Autodesk Fusion 360 part; units mm, degrees
(part 3 of 4)
sketch "Sketch9" plane through (0, 17, 0) normal (0, 1, 0) x (-1, 0, 0)
  line L0 (-96.2371, 19.0203) -> (-96.2371, 18.4195)
  line L1 (-96.2371, 18.4195) -> (-95.4378, 18.4195)
  line L2 (-95.4378, 18.4195) -> (-95.4378, 5.6203)
  line L3 (-95.4378, 5.6203) -> (-96.2371, 5.6203)
  line L4 (-96.2371, 5.6203) -> (-96.2371, 5.0195)
  line L5 (-96.2371, 5.0195) -> (-110.23659, 5.0195)
  line L6 (-110.23659, 5.0195) -> (-110.23659, 5.6203)
  line L7 (-110.23659, 5.6203) -> (-111.03722, 5.6203)
  line L8 (-111.03722, 5.6203) -> (-111.03722, 18.4195)
  line L9 (-111.03722, 18.4195) -> (-110.23659, 18.4195)
  line L10 (-110.23659, 18.4195) -> (-110.23659, 19.0203)
  line L11 (-110.23659, 19.0203) -> (-96.2371, 19.0203)
  line L12 (-31.1441, 18.4195) -> (-31.1441, 5.6203)
  line L13 (-31.1441, 5.6203) -> (-31.9449, 5.6203)
  line L14 (-31.9449, 5.6203) -> (-31.9449, 5.0195)
  line L15 (-31.9449, 5.0195) -> (-45.9442, 5.0195)
  line L16 (-45.9442, 5.0195) -> (-45.9442, 5.6203)
  line L17 (-45.9442, 5.6203) -> (-46.745, 5.6203)
  line L18 (-46.745, 5.6203) -> (-46.745, 18.4195)
  line L19 (-46.745, 18.4195) -> (-45.9442, 18.4195)
  line L20 (-45.9442, 18.4195) -> (-45.9442, 19.0203)
  line L21 (-45.9442, 19.0203) -> (-31.9449, 19.0203)
  line L22 (-31.9449, 19.0203) -> (-31.9449, 18.4195)
  line L23 (-31.9449, 18.4195) -> (-31.1441, 18.4195)
  line L24 (-21.6191, 24.6704) -> (-22.4199, 24.6704)
  line L25 (-22.4199, 24.6704) -> (-22.4199, 24.0696)
  line L26 (-22.4199, 24.0696) -> (-36.4192, 24.0696)
  line L27 (-36.4192, 24.0696) -> (-36.4192, 24.6704)
  line L28 (-36.4192, 24.6704) -> (-37.2186, 24.6704)
  line L29 (-37.2186, 24.6704) -> (-37.2186, 37.4695)
  line L30 (-37.2186, 37.4695) -> (-36.4192, 37.4695)
  line L31 (-36.4192, 37.4695) -> (-36.4192, 38.0703)
  line L32 (-36.4192, 38.0703) -> (-22.4199, 38.0703)
  line L33 (-22.4199, 38.0703) -> (-22.4199, 37.4695)
  line L34 (-22.4199, 37.4695) -> (-21.6191, 37.4695)
  line L35 (-21.6191, 37.4695) -> (-21.6191, 24.6704)
  line L36 (-62.6115, -0.0297) -> (-46.391293, -0.0297)
  line L37 (-46.391293, -0.0297) -> (-46.391293, -0.6305)
  line L38 (-46.391293, -0.6305) -> (-45.592293, -0.6305)
  line L39 (-45.592293, -0.6305) -> (-45.592293, -3.205101)
  line L40 (-45.592293, -3.205101) -> (-43.156293, -3.205101)
  arc A0 (-43.156293, -8.205101) -> (-43.156293, -3.205101) centre (-43.156293, -5.705101) ccw
  line L41 (-43.156293, -8.205101) -> (-45.592293, -8.205101)
  line L42 (-45.592293, -8.205101) -> (-45.592293, -13.42971)
  line L43 (-45.592293, -13.42971) -> (-46.391293, -13.42971)
  line L44 (-46.391293, -13.42971) -> (-46.391293, -14.03054)
  line L45 (-46.391293, -14.03054) -> (-62.6115, -14.03054)
  line L46 (-62.6115, -14.03054) -> (-62.6115, -13.42971)
  line L47 (-62.6115, -13.42971) -> (-63.4123, -13.42971)
  line L48 (-63.4123, -13.42971) -> (-63.4123, -0.6305)
  line L49 (-63.4123, -0.6305) -> (-62.6115, -0.6305)
  line L50 (-62.6115, -0.6305) -> (-62.6115, -0.0297)
  circle A1 centre (-90.056293, 5.844899) radius 2.5
  line L51 (-100.2003, -13.42971) -> (-100.9996, -13.42971)
  line L52 (-100.9996, -13.42971) -> (-100.9996, -14.03054)
  line L53 (-100.9996, -14.03054) -> (-115.00047, -14.03054)
  line L54 (-115.00047, -14.03054) -> (-115.00047, -14)
  line L55 (-115.00047, -14) -> (-117.382293, -14)
  line L56 (-117.382293, -14) -> (-117.382293, -13.42971)
  line L57 (-117.382293, -13.42971) -> (-118.181293, -13.42971)
  line L58 (-118.181293, -13.42971) -> (-118.181293, -0.6305)
  line L59 (-118.181293, -0.6305) -> (-117.382293, -0.6305)
  line L60 (-117.382293, -0.6305) -> (-117.382293, -0.0297)
  line L61 (-117.382293, -0.0297) -> (-100.9996, -0.0297)
  line L62 (-100.9996, -0.0297) -> (-100.9996, -0.6305)
  line L63 (-100.9996, -0.6305) -> (-100.2003, -0.6305)
  line L64 (-100.2003, -0.6305) -> (-100.2003, -13.42971)
  line L65 (120.457, 5.6203) -> (120.457, 5.0195)
  line L66 (120.457, 5.0195) -> (106.457, 5.0195)
  line L67 (106.457, 5.0195) -> (106.457, 5.6203)
  line L68 (106.457, 5.6203) -> (105.656, 5.6203)
  line L69 (105.656, 5.6203) -> (105.656, 18.4195)
  line L70 (105.656, 18.4195) -> (106.457, 18.4195)
  line L71 (106.457, 18.4195) -> (106.457, 19.0203)
  line L72 (106.457, 19.0203) -> (120.457, 19.0203)
  line L73 (120.457, 19.0203) -> (120.457, 18.4195)
  line L74 (120.457, 18.4195) -> (121.257, 18.4195)
  line L75 (121.257, 18.4195) -> (121.257, 5.6203)
  line L76 (121.257, 5.6203) -> (120.457, 5.6203)
  circle A2 centre (62.431, -5.905101) radius 2.5
  line L77 (99.313, 57.1203) -> (113.313, 57.1203)
  line L78 (113.313, 57.1203) -> (113.313, 56.5195)
  line L79 (113.313, 56.5195) -> (114.112, 56.5195)
  line L80 (114.112, 56.5195) -> (114.112, 43.7204)
  line L81 (114.112, 43.7204) -> (113.313, 43.7204)
  line L82 (113.313, 43.7204) -> (113.313, 43.1196)
  line L83 (113.313, 43.1196) -> (99.313, 43.1196)
  line L84 (99.313, 43.1196) -> (99.313, 43.7204)
  line L85 (99.313, 43.7204) -> (98.513, 43.7204)
  line L86 (98.513, 43.7204) -> (98.513, 56.5195)
  line L87 (98.513, 56.5195) -> (99.313, 56.5195)
  line L88 (99.313, 56.5195) -> (99.313, 57.1203)
  line L89 (101.693, 24.0696) -> (101.693, 24.6704)
  line L90 (101.693, 24.6704) -> (100.894, 24.6704)
  line L91 (100.894, 24.6704) -> (100.894, 37.4695)
  line L92 (100.894, 37.4695) -> (101.693, 37.4695)
  line L93 (101.693, 37.4695) -> (101.693, 38.0703)
  line L94 (101.693, 38.0703) -> (115.694, 38.0703)
  line L95 (115.694, 38.0703) -> (115.694, 37.4695)
  line L96 (115.694, 37.4695) -> (116.493, 37.4695)
  line L97 (116.493, 37.4695) -> (116.493, 24.6704)
  line L98 (116.493, 24.6704) -> (115.694, 24.6704)
  line L99 (115.694, 24.6704) -> (115.694, 24.0696)
  line L100 (115.694, 24.0696) -> (101.693, 24.0696)
  line L101 (87.119, 56.5195) -> (87.918, 56.5195)
  line L102 (87.918, 56.5195) -> (87.918, 43.7204)
  line L103 (87.918, 43.7204) -> (87.119, 43.7204)
  line L104 (87.119, 43.7204) -> (87.119, 43.1196)
  line L105 (87.119, 43.1196) -> (73.118, 43.1196)
  line L106 (73.118, 43.1196) -> (73.118, 43.7204)
  line L107 (73.118, 43.7204) -> (72.319, 43.7204)
  line L108 (72.319, 43.7204) -> (72.319, 56.5195)
  line L109 (72.319, 56.5195) -> (73.118, 56.5195)
  line L110 (73.118, 56.5195) -> (73.118, 57.1203)
  line L111 (73.118, 57.1203) -> (87.119, 57.1203)
  line L112 (87.119, 57.1203) -> (87.119, 56.5195)
  line L113 (87.407, 5.0195) -> (87.407, 5.6203)
  line L114 (87.407, 5.6203) -> (86.606, 5.6203)
  line L115 (86.606, 5.6203) -> (86.606, 18.4195)
  line L116 (86.606, 18.4195) -> (87.407, 18.4195)
  line L117 (87.407, 18.4195) -> (87.407, 19.0203)
  line L118 (87.407, 19.0203) -> (101.407, 19.0203)
  line L119 (101.407, 19.0203) -> (101.407, 18.4195)
  line L120 (101.407, 18.4195) -> (102.207, 18.4195)
  line L121 (102.207, 18.4195) -> (102.207, 5.6203)
  line L122 (102.207, 5.6203) -> (101.407, 5.6203)
  line L123 (101.407, 5.6203) -> (101.407, 5.0195)
  line L124 (101.407, 5.0195) -> (87.407, 5.0195)
  line L125 (77.882, 24.6704) -> (77.081, 24.6704)
  line L126 (77.081, 24.6704) -> (77.081, 37.4695)
  line L127 (77.081, 37.4695) -> (77.882, 37.4695)
  line L128 (77.882, 37.4695) -> (77.882, 38.0703)
  line L129 (77.882, 38.0703) -> (91.882, 38.0703)
  line L130 (91.882, 38.0703) -> (91.882, 37.4695)
  line L131 (91.882, 37.4695) -> (92.682, 37.4695)
  line L132 (92.682, 37.4695) -> (92.682, 24.6704)
  line L133 (92.682, 24.6704) -> (91.882, 24.6704)
  line L134 (91.882, 24.6704) -> (91.882, 24.0696)
  line L135 (91.882, 24.0696) -> (77.882, 24.0696)
  line L136 (77.882, 24.0696) -> (77.882, 24.6704)
  circle A3 centre (90.731, 42.8948) radius 2.5
  line L137 (121.257, -0.6305) -> (121.257, -13.42971)
  line L138 (121.257, -13.42971) -> (120.457, -13.42971)
  line L139 (120.457, -13.42971) -> (120.457, -14.03054)
  line L140 (120.457, -14.03054) -> (106.457, -14.03054)
  line L141 (106.457, -14.03054) -> (106.457, -14)
  line L142 (106.457, -14) -> (101.407, -14)
  line L143 (101.407, -14) -> (101.407, -14.03054)
  line L144 (101.407, -14.03054) -> (87.407, -14.03054)
  line L145 (87.407, -14.03054) -> (87.407, -13.42971)
  line L146 (87.407, -13.42971) -> (86.606, -13.42971)
  line L147 (86.606, -13.42971) -> (86.606, -0.6305)
  line L148 (86.606, -0.6305) -> (87.407, -0.6305)
  line L149 (87.407, -0.6305) -> (87.407, -0.0297)
  line L150 (87.407, -0.0297) -> (120.457, -0.0297)
  line L151 (120.457, -0.0297) -> (120.457, -0.6305)
  line L152 (120.457, -0.6305) -> (121.257, -0.6305)
  line L153 (41.363, -0.6305) -> (42.162, -0.6305)
  line L154 (42.162, -0.6305) -> (42.162, -0.0297)
  line L155 (42.162, -0.0297) -> (58.544, -0.0297)
  line L156 (58.544, -0.0297) -> (58.544, -0.6305)
  line L157 (58.544, -0.6305) -> (59.343, -0.6305)
  line L158 (59.343, -0.6305) -> (59.343, -13.42971)
  line L159 (59.343, -13.42971) -> (58.544, -13.42971)
  line L160 (58.544, -13.42971) -> (58.544, -14.03054)
  line L161 (58.544, -14.03054) -> (44.543, -14.03054)
  line L162 (44.543, -14.03054) -> (44.543, -14)
  line L163 (44.543, -14) -> (42.162, -14)
  line L164 (42.162, -14) -> (42.162, -13.42971)
  line L165 (42.162, -13.42971) -> (41.363, -13.42971)
  line L166 (41.363, -13.42971) -> (41.363, -0.6305)
  line L167 (25.205, 18.4195) -> (26.006, 18.4195)
  line L168 (26.006, 18.4195) -> (26.006, 5.6203)
  line L169 (26.006, 5.6203) -> (25.205, 5.6203)
  line L170 (25.205, 5.6203) -> (25.205, 5.0195)
  line L171 (25.205, 5.0195) -> (11.206, 5.0195)
  line L172 (11.206, 5.0195) -> (11.206, 5.6203)
  line L173 (11.206, 5.6203) -> (10.405, 5.6203)
  line L174 (10.405, 5.6203) -> (10.405, 18.4195)
  line L175 (10.405, 18.4195) -> (11.206, 18.4195)
  line L176 (11.206, 18.4195) -> (11.206, 19.0203)
  line L177 (11.206, 19.0203) -> (17.022586, 19.0203)
  line L178 (17.022586, 19.0203) -> (17.022586, 19.279382)
  arc A4 (19.339414, 19.279382) -> (17.022586, 19.279382) centre (18.181, 21.4948) ccw
  line L179 (19.339414, 19.279382) -> (19.339414, 19.0203)
  line L180 (19.339414, 19.0203) -> (25.205, 19.0203)
  line L181 (25.205, 19.0203) -> (25.205, 18.4195)
  line L182 (-100.2003, 24.6704) -> (-100.9996, 24.6704)
  line L183 (-100.9996, 24.6704) -> (-100.9996, 24.0696)
  line L184 (-100.9996, 24.0696) -> (-115.00047, 24.0696)
  line L185 (-115.00047, 24.0696) -> (-115.00047, 24.6704)
  line L186 (-115.00047, 24.6704) -> (-115.79972, 24.6704)
  line L187 (-115.79972, 24.6704) -> (-115.79972, 37.4695)
  line L188 (-115.79972, 37.4695) -> (-115.00047, 37.4695)
  line L189 (-115.00047, 37.4695) -> (-115.00047, 38.0703)
  line L190 (-115.00047, 38.0703) -> (-100.9996, 38.0703)
  line L191 (-100.9996, 38.0703) -> (-100.9996, 37.4695)
  line L192 (-100.9996, 37.4695) -> (-100.2003, 37.4695)
  line L193 (-100.2003, 37.4695) -> (-100.2003, 24.6704)
  line L194 (-102.5816, 43.7204) -> (-103.3808, 43.7204)
  line L195 (-103.3808, 43.7204) -> (-103.3808, 43.1196)
  line L196 (-103.3808, 43.1196) -> (-117.38173, 43.1196)
  line L197 (-117.38173, 43.1196) -> (-117.38173, 43.7204)
  line L198 (-117.38173, 43.7204) -> (-118.18099, 43.7204)
  line L199 (-118.18099, 43.7204) -> (-118.18099, 56.5195)
  line L200 (-118.18099, 56.5195) -> (-117.38173, 56.5195)
  line L201 (-117.38173, 56.5195) -> (-117.38173, 57.1203)
  line L202 (-117.38173, 57.1203) -> (-103.3808, 57.1203)
  line L203 (-103.3808, 57.1203) -> (-103.3808, 56.5195)
  line L204 (-103.3808, 56.5195) -> (-102.5816, 56.5195)
  line L205 (-102.5816, 56.5195) -> (-102.5816, 43.7204)
  line L206 (-98.372293, -13.42971) -> (-99.171293, -13.42971)
  line L207 (-99.171293, -13.42971) -> (-99.171293, -0.6305)
  line L208 (-99.171293, -0.6305) -> (-98.372293, -0.6305)
  line L209 (-98.372293, -0.6305) -> (-98.372293, 0)
  line L210 (-98.372293, 0) -> (-65.401293, 0)
  line L211 (-65.401293, 0) -> (-65.401293, -0.6305)
  line L212 (-65.401293, -0.6305) -> (-64.602293, -0.6305)
  line L213 (-64.602293, -0.6305) -> (-64.602293, -13.42971)
  line L214 (-64.602293, -13.42971) -> (-65.401293, -13.42971)
  line L215 (-65.401293, -13.42971) -> (-65.401293, -14.03054)
  line L216 (-65.401293, -14.03054) -> (-98.372293, -14.03054)
  line L217 (-98.372293, -14.03054) -> (-98.372293, -13.42971)
  line L218 (-60.5185, 38.0703) -> (-60.5185, 37.4695)
  line L219 (-60.5185, 37.4695) -> (-59.7177, 37.4695)
  line L220 (-59.7177, 37.4695) -> (-59.7177, 24.6704)
  line L221 (-59.7177, 24.6704) -> (-60.5185, 24.6704)
  line L222 (-60.5185, 24.6704) -> (-60.5185, 24.0696)
  line L223 (-60.5185, 24.0696) -> (-74.5178, 24.0696)
  line L224 (-74.5178, 24.0696) -> (-74.5178, 24.6704)
  line L225 (-74.5178, 24.6704) -> (-75.3186, 24.6704)
  line L226 (-75.3186, 24.6704) -> (-75.3186, 37.4695)
  line L227 (-75.3186, 37.4695) -> (-74.5178, 37.4695)
  line L228 (-74.5178, 37.4695) -> (-74.5178, 38.0703)
  line L229 (-74.5178, 38.0703) -> (-60.5185, 38.0703)
  line L230 (-87.582873, 38.0703) -> (-79.5699, 38.0703)
  line L231 (-79.5699, 38.0703) -> (-79.5699, 37.4695)
  line L232 (-79.5699, 37.4695) -> (-78.7691, 37.4695)
  line L233 (-78.7691, 37.4695) -> (-78.7691, 24.6704)
  line L234 (-78.7691, 24.6704) -> (-79.5699, 24.6704)
  line L235 (-79.5699, 24.6704) -> (-79.5699, 24.0696)
  line L236 (-79.5699, 24.0696) -> (-93.5692, 24.0696)
  line L237 (-93.5692, 24.0696) -> (-93.5692, 24.6704)
  line L238 (-93.5692, 24.6704) -> (-94.3699, 24.6704)
  line L239 (-94.3699, 24.6704) -> (-94.3699, 37.4695)
  line L240 (-94.3699, 37.4695) -> (-93.5692, 37.4695)
  line L241 (-93.5692, 37.4695) -> (-93.5692, 38.0703)
  line L242 (-93.5692, 38.0703) -> (-89.429714, 38.0703)
  line L243 (-89.429714, 38.0703) -> (-89.429714, 38.271592)
  arc A5 (-89.429714, 42.918008) -> (-89.429714, 38.271592) centre (-88.506293, 40.5948) ccw
  line L244 (-89.429714, 42.918008) -> (-89.429714, 43.1196)
  line L245 (-89.429714, 43.1196) -> (-98.3317, 43.1196)
  line L246 (-98.3317, 43.1196) -> (-98.3317, 43.7204)
  line L247 (-98.3317, 43.7204) -> (-99.131, 43.7204)
  line L248 (-99.131, 43.7204) -> (-99.131, 56.5195)
  line L249 (-99.131, 56.5195) -> (-98.3317, 56.5195)
  line L250 (-98.3317, 56.5195) -> (-98.3317, 57.1203)
  line L251 (-98.3317, 57.1203) -> (-84.331, 57.1203)
  line L252 (-84.331, 57.1203) -> (-84.331, 56.5195)
  line L253 (-84.331, 56.5195) -> (-83.5316, 56.5195)
  line L254 (-83.5316, 56.5195) -> (-83.5316, 43.7204)
  line L255 (-83.5316, 43.7204) -> (-84.331, 43.7204)
  line L256 (-84.331, 43.7204) -> (-84.331, 43.1196)
  line L257 (-84.331, 43.1196) -> (-87.582873, 43.1196)
  line L258 (-87.582873, 43.1196) -> (-87.582873, 42.918008)
  arc A6 (-87.582873, 38.271592) -> (-87.582873, 42.918008) centre (-88.506293, 40.5948) ccw
  line L259 (-87.582873, 38.271592) -> (-87.582873, 38.0703)
  line L260 (-27.695, 5.6203) -> (-27.695, 18.4195)
  line L261 (-27.695, 18.4195) -> (-26.8942, 18.4195)
  line L262 (-26.8942, 18.4195) -> (-26.8942, 19.0203)
  line L263 (-26.8942, 19.0203) -> (-12.895, 19.0203)
  line L264 (-12.895, 19.0203) -> (-12.895, 18.4195)
  line L265 (-12.895, 18.4195) -> (-12.094, 18.4195)
  line L266 (-12.094, 18.4195) -> (-12.094, 5.6203)
  line L267 (-12.094, 5.6203) -> (-12.895, 5.6203)
  line L268 (-12.895, 5.6203) -> (-12.895, 5.0195)
  line L269 (-12.895, 5.0195) -> (-26.8942, 5.0195)
  line L270 (-26.8942, 5.0195) -> (-26.8942, 5.6203)
  line L271 (-26.8942, 5.6203) -> (-27.695, 5.6203)
  arc A7 (-13.437968, 42.823995) -> (-13.437968, 38.365605) centre (-12.306293, 40.5948) ccw
  line L272 (-13.437968, 42.823995) -> (-13.437968, 43.1196)
  line L273 (-13.437968, 43.1196) -> (-22.1317, 43.1196)
  line L274 (-22.1317, 43.1196) -> (-22.1317, 43.7204)
  line L275 (-22.1317, 43.7204) -> (-22.9311, 43.7204)
  line L276 (-22.9311, 43.7204) -> (-22.9311, 56.5195)
  line L277 (-22.9311, 56.5195) -> (-22.1317, 56.5195)
  line L278 (-22.1317, 56.5195) -> (-22.1317, 57.1203)
  line L279 (-22.1317, 57.1203) -> (-8.131, 57.1203)
  line L280 (-8.131, 57.1203) -> (-8.131, 56.5195)
  line L281 (-8.131, 56.5195) -> (-7.332, 56.5195)
  line L282 (-7.332, 56.5195) -> (-7.332, 43.7204)
  line L283 (-7.332, 43.7204) -> (-8.131, 43.7204)
  line L284 (-8.131, 43.7204) -> (-8.131, 43.1196)
  line L285 (-8.131, 43.1196) -> (-11.174619, 43.1196)
  line L286 (-11.174619, 43.1196) -> (-11.174619, 42.823995)
  arc A8 (-11.174619, 38.365605) -> (-11.174619, 42.823995) centre (-12.306293, 40.5948) ccw
  line L287 (-11.174619, 38.365605) -> (-11.174619, 38.0703)
  line L288 (-11.174619, 38.0703) -> (-3.37, 38.0703)
  line L289 (-3.37, 38.0703) -> (-3.37, 37.4695)
  line L290 (-3.37, 37.4695) -> (-2.569, 37.4695)
  line L291 (-2.569, 37.4695) -> (-2.569, 24.6704)
  line L292 (-2.569, 24.6704) -> (-3.37, 24.6704)
  line L293 (-3.37, 24.6704) -> (-3.37, 24.0696)
  line L294 (-3.37, 24.0696) -> (-17.369, 24.0696)
  line L295 (-17.369, 24.0696) -> (-17.369, 24.6704)
  line L296 (-17.369, 24.6704) -> (-18.17, 24.6704)
  line L297 (-18.17, 24.6704) -> (-18.17, 37.4695)
  line L298 (-18.17, 37.4695) -> (-17.369, 37.4695)
  line L299 (-17.369, 37.4695) -> (-17.369, 38.0703)
  line L300 (-17.369, 38.0703) -> (-13.437968, 38.0703)
  line L301 (-13.437968, 38.0703) -> (-13.437968, 38.365605)
  line L302 (68.069, 56.5195) -> (68.868, 56.5195)
  line L303 (68.868, 56.5195) -> (68.868, 43.7204)
  line L304 (68.868, 43.7204) -> (68.069, 43.7204)
  line L305 (68.069, 43.7204) -> (68.069, 43.1196)
  line L306 (68.069, 43.1196) -> (54.068, 43.1196)
  line L307 (54.068, 43.1196) -> (54.068, 43.7204)
  line L308 (54.068, 43.7204) -> (53.269, 43.7204)
  line L309 (53.269, 43.7204) -> (53.269, 56.5195)
  line L310 (53.269, 56.5195) -> (54.068, 56.5195)
  line L311 (54.068, 56.5195) -> (54.068, 57.1203)
  line L312 (54.068, 57.1203) -> (68.069, 57.1203)
  line L313 (68.069, 57.1203) -> (68.069, 56.5195)
  line L314 (67.556, -0.6305) -> (68.357, -0.6305)
  line L315 (68.357, -0.6305) -> (68.357, -0.0297)
  line L316 (68.357, -0.0297) -> (82.357, -0.0297)
  line L317 (82.357, -0.0297) -> (82.357, -0.6305)
  line L318 (82.357, -0.6305) -> (83.157, -0.6305)
  line L319 (83.157, -0.6305) -> (83.157, -13.42971)
  line L320 (83.157, -13.42971) -> (82.357, -13.42971)
  line L321 (82.357, -13.42971) -> (82.357, -14.03054)
  line L322 (82.357, -14.03054) -> (68.357, -14.03054)
  line L323 (68.357, -14.03054) -> (68.357, -13.42971)
  line L324 (68.357, -13.42971) -> (67.556, -13.42971)
  line L325 (67.556, -13.42971) -> (67.556, -0.6305)
  line L326 (68.357, 5.0195) -> (68.357, 5.6203)
  line L327 (68.357, 5.6203) -> (67.556, 5.6203)
  line L328 (67.556, 5.6203) -> (67.556, 18.4195)
  line L329 (67.556, 18.4195) -> (68.357, 18.4195)
  line L330 (68.357, 18.4195) -> (68.357, 19.0203)
  line L331 (68.357, 19.0203) -> (82.357, 19.0203)
  line L332 (82.357, 19.0203) -> (82.357, 18.4195)
  line L333 (82.357, 18.4195) -> (83.157, 18.4195)
  line L334 (83.157, 18.4195) -> (83.157, 5.6203)
  line L335 (83.157, 5.6203) -> (82.357, 5.6203)
  line L336 (82.357, 5.6203) -> (82.357, 5.0195)
  line L337 (82.357, 5.0195) -> (68.357, 5.0195)
  line L338 (-79.2817, 56.5195) -> (-79.2817, 57.1203)
  line L339 (-79.2817, 57.1203) -> (-65.281, 57.1203)
  line L340 (-65.281, 57.1203) -> (-65.281, 56.5195)
  line L341 (-65.281, 56.5195) -> (-64.4816, 56.5195)
  line L342 (-64.4816, 56.5195) -> (-64.4816, 43.7204)
  line L343 (-64.4816, 43.7204) -> (-65.281, 43.7204)
  line L344 (-65.281, 43.7204) -> (-65.281, 43.1196)
  line L345 (-65.281, 43.1196) -> (-79.2817, 43.1196)
  line L346 (-79.2817, 43.1196) -> (-79.2817, 43.7204)
  line L347 (-79.2817, 43.7204) -> (-80.0811, 43.7204)
  line L348 (-80.0811, 43.7204) -> (-80.0811, 56.5195)
  line L349 (-80.0811, 56.5195) -> (-79.2817, 56.5195)
  line L350 (-70.0449, 5.0195) -> (-84.0442, 5.0195)
  line L351 (-84.0442, 5.0195) -> (-84.0442, 5.6203)
  line L352 (-84.0442, 5.6203) -> (-84.8449, 5.6203)
  line L353 (-84.8449, 5.6203) -> (-84.8449, 18.4195)
  line L354 (-84.8449, 18.4195) -> (-84.0442, 18.4195)
  line L355 (-84.0442, 18.4195) -> (-84.0442, 19.0203)
  line L356 (-84.0442, 19.0203) -> (-70.0449, 19.0203)
  line L357 (-70.0449, 19.0203) -> (-70.0449, 18.4195)
  line L358 (-70.0449, 18.4195) -> (-69.2441, 18.4195)
  line L359 (-69.2441, 18.4195) -> (-69.2441, 5.6203)
  line L360 (-69.2441, 5.6203) -> (-70.0449, 5.6203)
  line L361 (-70.0449, 5.6203) -> (-70.0449, 5.0195)
  line L362 (-50.1941, 5.6203) -> (-50.9949, 5.6203)
  line L363 (-50.9949, 5.6203) -> (-50.9949, 5.0195)
  line L364 (-50.9949, 5.0195) -> (-64.9942, 5.0195)
  line L365 (-64.9942, 5.0195) -> (-64.9942, 5.6203)
  line L366 (-64.9942, 5.6203) -> (-65.795, 5.6203)
  line L367 (-65.795, 5.6203) -> (-65.795, 18.4195)
  line L368 (-65.795, 18.4195) -> (-64.9942, 18.4195)
  line L369 (-64.9942, 18.4195) -> (-64.9942, 19.0203)
  line L370 (-64.9942, 19.0203) -> (-50.9949, 19.0203)
  line L371 (-50.9949, 19.0203) -> (-50.9949, 18.4195)
  line L372 (-50.9949, 18.4195) -> (-50.1941, 18.4195)
  line L373 (-50.1941, 18.4195) -> (-50.1941, 5.6203)
  line L374 (35.532, 37.4695) -> (35.532, 24.6704)
  line L375 (35.532, 24.6704) -> (34.732, 24.6704)
  line L376 (34.732, 24.6704) -> (34.732, 24.0696)
  line L377 (34.732, 24.0696) -> (20.732, 24.0696)
  line L378 (20.732, 24.0696) -> (20.732, 24.6704)
  line L379 (20.732, 24.6704) -> (19.931, 24.6704)
  line L380 (19.931, 24.6704) -> (19.931, 37.4695)
  line L381 (19.931, 37.4695) -> (20.732, 37.4695)
  line L382 (20.732, 37.4695) -> (20.732, 38.0703)
  line L383 (20.732, 38.0703) -> (34.732, 38.0703)
  line L384 (34.732, 38.0703) -> (34.732, 37.4695)
  line L385 (34.732, 37.4695) -> (35.532, 37.4695)
  line L386 (15.682, 38.0703) -> (15.682, 37.4695)
  line L387 (15.682, 37.4695) -> (16.482, 37.4695)
  line L388 (16.482, 37.4695) -> (16.482, 24.6704)
  line L389 (16.482, 24.6704) -> (15.682, 24.6704)
  line L390 (15.682, 24.6704) -> (15.682, 24.0696)
  line L391 (15.682, 24.0696) -> (1.682, 24.0696)
  line L392 (1.682, 24.0696) -> (1.682, 24.6704)
  line L393 (1.682, 24.6704) -> (0.881, 24.6704)
  line L394 (0.881, 24.6704) -> (0.881, 37.4695)
  line L395 (0.881, 37.4695) -> (1.682, 37.4695)
  line L396 (1.682, 37.4695) -> (1.682, 38.0703)
  line L397 (1.682, 38.0703) -> (15.682, 38.0703)
  line L398 (-61.0311, 56.5195) -> (-60.2317, 56.5195)
  line L399 (-60.2317, 56.5195) -> (-60.2317, 57.1203)
  line L400 (-60.2317, 57.1203) -> (-46.231, 57.1203)
  line L401 (-46.231, 57.1203) -> (-46.231, 56.5195)
  line L402 (-46.231, 56.5195) -> (-45.4316, 56.5195)
  line L403 (-45.4316, 56.5195) -> (-45.4316, 43.7204)
  line L404 (-45.4316, 43.7204) -> (-46.231, 43.7204)
  line L405 (-46.231, 43.7204) -> (-46.231, 43.1196)
  line L406 (-46.231, 43.1196) -> (-60.2317, 43.1196)
  line L407 (-60.2317, 43.1196) -> (-60.2317, 43.7204)
  line L408 (-60.2317, 43.7204) -> (-61.0311, 43.7204)
  line L409 (-61.0311, 43.7204) -> (-61.0311, 56.5195)
  line L410 (10.919, 43.7204) -> (10.919, 43.1196)
  line L411 (10.919, 43.1196) -> (-3.082, 43.1196)
  line L412 (-3.082, 43.1196) -> (-3.082, 43.7204)
  line L413 (-3.082, 43.7204) -> (-3.881, 43.7204)
  line L414 (-3.881, 43.7204) -> (-3.881, 56.5195)
  line L415 (-3.881, 56.5195) -> (-3.082, 56.5195)
  line L416 (-3.082, 56.5195) -> (-3.082, 57.1203)
  line L417 (-3.082, 57.1203) -> (10.919, 57.1203)
  line L418 (10.919, 57.1203) -> (10.919, 56.5195)
  line L419 (10.919, 56.5195) -> (11.718, 56.5195)
  line L420 (11.718, 56.5195) -> (11.718, 43.7204)
  line L421 (11.718, 43.7204) -> (10.919, 43.7204)
  line L422 (26.782, -2.3007) -> (26.782, -1.3)
  line L423 (26.782, -1.3) -> (28.507, -1.3)
  line L424 (28.507, -1.3) -> (28.507, -0.1795)
  line L425 (28.507, -0.1795) -> (31.806, -0.1795)
  line L426 (31.806, -0.1795) -> (31.806, -1.3)
  line L427 (31.806, -1.3) -> (33.432, -1.3)
  line L428 (33.432, -1.3) -> (33.432, -4.7302)
  line L429 (33.432, -4.7302) -> (34.307, -4.7302)
  line L430 (34.307, -4.7302) -> (34.307, -7.53034)
  line L431 (34.307, -7.53034) -> (33.432, -7.53034)
  line L432 (33.432, -7.53034) -> (33.432, -14.0004)
  line L433 (33.432, -14.0004) -> (31.806, -14.0004)
  line L434 (31.806, -14.0004) -> (31.806, -14.78019)
  line L435 (31.806, -14.78019) -> (28.507, -14.78019)
  line L436 (28.507, -14.78019) -> (28.507, -14.0004)
  line L437 (28.507, -14.0004) -> (26.782, -14.0004)
  line L438 (26.782, -14.0004) -> (26.782, -12.99978)
  line L439 (26.782, -12.99978) -> (26.007, -12.99978)
  line L440 (26.007, -12.99978) -> (26.007, -13.42971)
  line L441 (26.007, -13.42971) -> (25.207, -13.42971)
  line L442 (25.207, -13.42971) -> (25.207, -14.03054)
  line L443 (25.207, -14.03054) -> (11.207, -14.03054)
  line L444 (11.207, -14.03054) -> (11.207, -13.42971)
  line L445 (11.207, -13.42971) -> (10.405, -13.42971)
  line L446 (10.405, -13.42971) -> (10.405, -12.99978)
  line L447 (10.405, -12.99978) -> (9.632, -12.99978)
  line L448 (9.632, -12.99978) -> (9.632, -14.0004)
  line L449 (9.632, -14.0004) -> (7.905, -14.0004)
  line L450 (7.905, -14.0004) -> (7.905, -14.78019)
  line L451 (7.905, -14.78019) -> (4.606, -14.78019)
  line L452 (4.606, -14.78019) -> (4.606, -14.0004)
  line L453 (4.606, -14.0004) -> (2.982, -14.0004)
  line L454 (2.982, -14.0004) -> (2.982, -7.53034)
  line L455 (2.982, -7.53034) -> (2.107, -7.53034)
  line L456 (2.107, -7.53034) -> (2.107, -4.7302)
  line L457 (2.107, -4.7302) -> (2.982, -4.7302)
  line L458 (2.982, -4.7302) -> (2.982, -1.3)
  line L459 (2.982, -1.3) -> (4.606, -1.3)
  line L460 (4.606, -1.3) -> (4.606, -0.1795)
  line L461 (4.606, -0.1795) -> (7.905, -0.1795)
  line L462 (7.905, -0.1795) -> (7.905, -1.3)
  line L463 (7.905, -1.3) -> (9.632, -1.3)
  line L464 (9.632, -1.3) -> (9.632, -2.3007)
  line L465 (9.632, -2.3007) -> (10.405, -2.3007)
  line L466 (10.405, -2.3007) -> (10.405, -0.6305)
  line L467 (10.405, -0.6305) -> (11.207, -0.6305)
  line L468 (11.207, -0.6305) -> (11.207, -0.0297)
  line L469 (11.207, -0.0297) -> (25.207, -0.0297)
  line L470 (25.207, -0.0297) -> (25.207, -0.6305)
  line L471 (25.207, -0.6305) -> (26.007, -0.6305)
  line L472 (26.007, -0.6305) -> (26.007, -2.3007)
  line L473 (26.007, -2.3007) -> (26.782, -2.3007)
  line L474 (-30.8506, -12.99978) -> (-30.8506, -14.0004)
  line L475 (-30.8506, -14.0004) -> (-32.576, -14.0004)
  line L476 (-32.576, -14.0004) -> (-32.576, -14.78019)
  line L477 (-32.576, -14.78019) -> (-35.8748, -14.78019)
  line L478 (-35.8748, -14.78019) -> (-35.8748, -14.0004)
  line L479 (-35.8748, -14.0004) -> (-37.4997, -14.0004)
  line L480 (-37.4997, -14.0004) -> (-37.4997, -7.53034)
  line L481 (-37.4997, -7.53034) -> (-38.3746, -7.53034)
  line L482 (-38.3746, -7.53034) -> (-38.3746, -4.7302)
  line L483 (-38.3746, -4.7302) -> (-37.4997, -4.7302)
  line L484 (-37.4997, -4.7302) -> (-37.4997, -1.3)
  line L485 (-37.4997, -1.3) -> (-35.8748, -1.3)
  line L486 (-35.8748, -1.3) -> (-35.8748, -0.1795)
  line L487 (-35.8748, -0.1795) -> (-32.576, -0.1795)
  line L488 (-32.576, -0.1795) -> (-32.576, -1.3)
  line L489 (-32.576, -1.3) -> (-30.8506, -1.3)
  line L490 (-30.8506, -1.3) -> (-30.8506, -2.3007)
  line L491 (-30.8506, -2.3007) -> (-30.0748, -2.3007)
  line L492 (-30.0748, -2.3007) -> (-30.0748, -0.6305)
  line L493 (-30.0748, -0.6305) -> (-29.2754, -0.6305)
  line L494 (-29.2754, -0.6305) -> (-29.2754, -0.0297)
  line L495 (-29.2754, -0.0297) -> (-15.275, -0.0297)
  line L496 (-15.275, -0.0297) -> (-15.275, -0.6305)
  line L497 (-15.275, -0.6305) -> (-14.475, -0.6305)
  line L498 (-14.475, -0.6305) -> (-14.475, -2.3007)
  line L499 (-14.475, -2.3007) -> (-13.701, -2.3007)
  line L500 (-13.701, -2.3007) -> (-13.701, -1.3)
  line L501 (-13.701, -1.3) -> (-11.976, -1.3)
  line L502 (-11.976, -1.3) -> (-11.976, -0.1795)
  line L503 (-11.976, -0.1795) -> (-8.675, -0.1795)
  line L504 (-8.675, -0.1795) -> (-8.675, -1.3)
  line L505 (-8.675, -1.3) -> (-7.05, -1.3)
  line L506 (-7.05, -1.3) -> (-7.05, -4.7302)
  line L507 (-7.05, -4.7302) -> (-6.176, -4.7302)
  line L508 (-6.176, -4.7302) -> (-6.176, -7.53034)
  line L509 (-6.176, -7.53034) -> (-7.05, -7.53034)
  line L510 (-7.05, -7.53034) -> (-7.05, -14.0004)
  line L511 (-7.05, -14.0004) -> (-8.675, -14.0004)
  line L512 (-8.675, -14.0004) -> (-8.675, -14.78019)
  line L513 (-8.675, -14.78019) -> (-11.976, -14.78019)
  line L514 (-11.976, -14.78019) -> (-11.976, -14.0004)
  line L515 (-11.976, -14.0004) -> (-13.701, -14.0004)
  line L516 (-13.701, -14.0004) -> (-13.701, -12.99978)
  line L517 (-13.701, -12.99978) -> (-14.475, -12.99978)
  line L518 (-14.475, -12.99978) -> (-14.475, -13.42971)
  line L519 (-14.475, -13.42971) -> (-15.275, -13.42971)
  line L520 (-15.275, -13.42971) -> (-15.275, -14.03054)
  line L521 (-15.275, -14.03054) -> (-29.2754, -14.03054)
  line L522 (-29.2754, -14.03054) -> (-29.2754, -13.42971)
  line L523 (-29.2754, -13.42971) -> (-30.0748, -13.42971)
  line L524 (-30.0748, -13.42971) -> (-30.0748, -12.99978)
  line L525 (-30.0748, -12.99978) -> (-30.8506, -12.99978)
  line L526 (-41.4685, 24.6704) -> (-41.4685, 24.0696)
  line L527 (-41.4685, 24.0696) -> (-55.4678, 24.0696)
  line L528 (-55.4678, 24.0696) -> (-55.4678, 24.6704)
  line L529 (-55.4678, 24.6704) -> (-56.2686, 24.6704)
  line L530 (-56.2686, 24.6704) -> (-56.2686, 37.4695)
  line L531 (-56.2686, 37.4695) -> (-55.4678, 37.4695)
  line L532 (-55.4678, 37.4695) -> (-55.4678, 38.0703)
  line L533 (-55.4678, 38.0703) -> (-41.4685, 38.0703)
  line L534 (-41.4685, 38.0703) -> (-41.4685, 37.4695)
  line L535 (-41.4685, 37.4695) -> (-40.6691, 37.4695)
  line L536 (-40.6691, 37.4695) -> (-40.6691, 24.6704)
  line L537 (-40.6691, 24.6704) -> (-41.4685, 24.6704)
  line L538 (49.019, 57.1203) -> (49.019, 56.5195)
  line L539 (49.019, 56.5195) -> (49.818, 56.5195)
  line L540 (49.818, 56.5195) -> (49.818, 43.7204)
  line L541 (49.818, 43.7204) -> (49.019, 43.7204)
  line L542 (49.019, 43.7204) -> (49.019, 43.1196)
  line L543 (49.019, 43.1196) -> (35.018, 43.1196)
  line L544 (35.018, 43.1196) -> (35.018, 43.7204)
  line L545 (35.018, 43.7204) -> (34.219, 43.7204)
  line L546 (34.219, 43.7204) -> (34.219, 56.5195)
  line L547 (34.219, 56.5195) -> (35.018, 56.5195)
  line L548 (35.018, 56.5195) -> (35.018, 57.1203)
  line L549 (35.018, 57.1203) -> (49.019, 57.1203)
  line L550 (15.968, 43.1196) -> (15.968, 43.7204)
  line L551 (15.968, 43.7204) -> (15.169, 43.7204)
  line L552 (15.169, 43.7204) -> (15.169, 56.5195)
  line L553 (15.169, 56.5195) -> (15.968, 56.5195)
  line L554 (15.968, 56.5195) -> (15.968, 57.1203)
  line L555 (15.968, 57.1203) -> (29.969, 57.1203)
  line L556 (29.969, 57.1203) -> (29.969, 56.5195)
  line L557 (29.969, 56.5195) -> (30.768, 56.5195)
  line L558 (30.768, 56.5195) -> (30.768, 43.7204)
  line L559 (30.768, 43.7204) -> (29.969, 43.7204)
  line L560 (29.969, 43.7204) -> (29.969, 43.1196)
  line L561 (29.969, 43.1196) -> (15.968, 43.1196)
  line L562 (-27.181, 43.1196) -> (-41.1817, 43.1196)
  line L563 (-41.1817, 43.1196) -> (-41.1817, 43.7204)
  line L564 (-41.1817, 43.7204) -> (-41.9811, 43.7204)
  line L565 (-41.9811, 43.7204) -> (-41.9811, 56.5195)
  line L566 (-41.9811, 56.5195) -> (-41.1817, 56.5195)
  line L567 (-41.1817, 56.5195) -> (-41.1817, 57.1203)
  line L568 (-41.1817, 57.1203) -> (-27.181, 57.1203)
  line L569 (-27.181, 57.1203) -> (-27.181, 56.5195)
  line L570 (-27.181, 56.5195) -> (-26.3816, 56.5195)
  line L571 (-26.3816, 56.5195) -> (-26.3816, 43.7204)
  line L572 (-26.3816, 43.7204) -> (-27.181, 43.7204)
  line L573 (-27.181, 43.7204) -> (-27.181, 43.1196)
  line L574 (45.057, 5.6203) -> (44.255, 5.6203)
  line L575 (44.255, 5.6203) -> (44.255, 5.0195)
  line L576 (44.255, 5.0195) -> (30.256, 5.0195)
  line L577 (30.256, 5.0195) -> (30.256, 5.6203)
  line L578 (30.256, 5.6203) -> (29.455, 5.6203)
  line L579 (29.455, 5.6203) -> (29.455, 18.4195)
  line L580 (29.455, 18.4195) -> (30.256, 18.4195)
  line L581 (30.256, 18.4195) -> (30.256, 19.0203)
  line L582 (30.256, 19.0203) -> (44.255, 19.0203)
  line L583 (44.255, 19.0203) -> (44.255, 18.4195)
  line L584 (44.255, 18.4195) -> (45.057, 18.4195)
  line L585 (45.057, 18.4195) -> (45.057, 5.6203)
  line L586 (-7.844, 19.0203) -> (6.155, 19.0203)
  line L587 (6.155, 19.0203) -> (6.155, 18.4195)
  line L588 (6.155, 18.4195) -> (6.956, 18.4195)
  line L589 (6.956, 18.4195) -> (6.956, 5.6203)
  line L590 (6.956, 5.6203) -> (6.155, 5.6203)
  line L591 (6.155, 5.6203) -> (6.155, 5.0195)
  line L592 (6.155, 5.0195) -> (-7.844, 5.0195)
  line L593 (-7.844, 5.0195) -> (-7.844, 5.6203)
  line L594 (-7.844, 5.6203) -> (-8.645, 5.6203)
  line L595 (-8.645, 5.6203) -> (-8.645, 18.4195)
  line L596 (-8.645, 18.4195) -> (-7.844, 18.4195)
  line L597 (-7.844, 18.4195) -> (-7.844, 19.0203)
  line L598 (58.031, 37.4695) -> (58.832, 37.4695)
  line L599 (58.832, 37.4695) -> (58.832, 38.0703)
  line L600 (58.832, 38.0703) -> (72.832, 38.0703)
  line L601 (72.832, 38.0703) -> (72.832, 37.4695)
  line L602 (72.832, 37.4695) -> (73.632, 37.4695)
  line L603 (73.632, 37.4695) -> (73.632, 24.6704)
  line L604 (73.632, 24.6704) -> (72.832, 24.6704)
  line L605 (72.832, 24.6704) -> (72.832, 24.0696)
  line L606 (72.832, 24.0696) -> (58.832, 24.0696)
  line L607 (58.832, 24.0696) -> (58.832, 24.6704)
  line L608 (58.832, 24.6704) -> (58.031, 24.6704)
  line L609 (58.031, 24.6704) -> (58.031, 37.4695)
  line L610 (38.981, 37.4695) -> (39.782, 37.4695)
  line L611 (39.782, 37.4695) -> (39.782, 38.0703)
  line L612 (39.782, 38.0703) -> (53.782, 38.0703)
  line L613 (53.782, 38.0703) -> (53.782, 37.4695)
  line L614 (53.782, 37.4695) -> (54.582, 37.4695)
  line L615 (54.582, 37.4695) -> (54.582, 24.6704)
  line L616 (54.582, 24.6704) -> (53.782, 24.6704)
  line L617 (53.782, 24.6704) -> (53.782, 24.0696)
  line L618 (53.782, 24.0696) -> (39.782, 24.0696)
  line L619 (39.782, 24.0696) -> (39.782, 24.6704)
  line L620 (39.782, 24.6704) -> (38.981, 24.6704)
  line L621 (38.981, 24.6704) -> (38.981, 37.4695)
  line L622 (63.307, 18.4195) -> (64.107, 18.4195)
  line L623 (64.107, 18.4195) -> (64.107, 5.6203)
  line L624 (64.107, 5.6203) -> (63.307, 5.6203)
  line L625 (63.307, 5.6203) -> (63.307, 5.0195)
  line L626 (63.307, 5.0195) -> (49.307, 5.0195)
  line L627 (49.307, 5.0195) -> (49.307, 5.6203)
  line L628 (49.307, 5.6203) -> (48.505, 5.6203)
  line L629 (48.505, 5.6203) -> (48.505, 18.4195)
  line L630 (48.505, 18.4195) -> (49.307, 18.4195)
  line L631 (49.307, 18.4195) -> (49.307, 19.0203)
  line L632 (49.307, 19.0203) -> (63.307, 19.0203)
  line L633 (63.307, 19.0203) -> (63.307, 18.4195)
  line L634 (-117.156293, -16.555101) -> (120.231, -16.555101)
  arc A9 (120.231, -16.555101) -> (123.231, -13.555101) centre (120.231, -13.555101) ccw
  line L635 (123.231, -13.555101) -> (123.231, 56.6448)
  arc A10 (123.231, 56.6448) -> (120.231, 59.6448) centre (120.231, 56.6448) ccw
  line L636 (120.231, 59.6448) -> (-117.156293, 59.6448)
  arc A11 (-117.156293, 59.6448) -> (-120.156293, 56.6448) centre (-117.156293, 56.6448) ccw
  line L637 (-120.156293, 56.6448) -> (-120.156293, -13.555101)
  arc A12 (-120.156293, -13.555101) -> (-117.156293, -16.555101) centre (-117.156293, -13.555101) ccw
extrude "Extrude5" add sketch "Sketch9" along normal blind 2 separate body contours L0 L1 L2 L3 L4 L5 L6 L7 L8 L9 L10 L11 | L12 L13 L14 L15 L16 L17 L18 L19 L20 L21 L22 L23 | L24 L25 L26 L27 L28 L29 L30 L31 L32 L33 L34 L35 | L36 L37 L38 L39 L40 A0 L41 L42 L43 L44 L45 L46 L47 L48 L49 L50 | A1 | L51 L52 L53 L54 L55 L56 L57 L58 L59 L60 L61 L62 L63 L64 | L65 L66 L67 L68 L69 L70 L71 L72 L73 L74 L75 L76 | A2 | L77 L78 L79 L80 L81 L82 L83 L84 L85 L86 L87 L88 | L89 L90 L91 L92 L93 L94 L95 L96 L97 L98 L99 L100 | L101 L102 L103 L104 L105 L106 L107 L108 L109 L110 L111 L112 | L113 L114 L115 L116 L117 L118 L119 L120 L121 L122 L123 L124 | L125 L126 L127 L128 L129 L130 L131 L132 L133 L134 L135 L136 | A3 | L137 L138 L139 L140 L141 L142 L143 L144 L145 L146 L147 L148 L149 L150 L151 L152 | L153 L154 L155 L156 L157 L158 L159 L160 L161 L162 L163 L164 L165 L166 | L167 L168 L169 L170 L171 L172 L173 L174 L175 L176 L177 L178 A4 L179 L180 L181 | L182 L183 L184 L185 L186 L187 L188 L189 L190 L191 L192 L193 | L194 L195 L196 L197 L198 L199 L200 L201 L202 L203 L204 L205 | L206 L207 L208 L209 L210 L211 L212 L213 L214 L215 L216 L217 | L218 L219 L220 L221 L222 L223 L224 L225 L226 L227 L228 L229 | L230 L231 L232 L233 L234 L235 L236 L237 L238 L239 L240 L241 L242 L243 A5 L244 L245 L246 L247 L248 L249 L250 L251 L252 L253 L254 L255 L256 L257 L258 A6 L259 | L260 L261 L262 L263 L264 L265 L266 L267 L268 L269 L270 L271 | A7 L272 L273 L274 L275 L276 L277 L278 L279 L280 L281 L282 L283 L284 L285 L286 A8 L287 L288 L289 L290 L291 L292 L293 L294 L295 L296 L297 L298 L299 L300 L301 | L302 L303 L304 L305 L306 L307 L308 L309 L310 L311 L312 L313 | L314 L315 L316 L317 L318 L319 L320 L321 L322 L323 L324 L325 | L326 L327 L328 L329 L330 L331 L332 L333 L334 L335 L336 L337 | L338 L339 L340 L341 L342 L343 L344 L345 L346 L347 L348 L349 | L350 L351 L352 L353 L354 L355 L356 L357 L358 L359 L360 L361 | L362 L363 L364 L365 L366 L367 L368 L369 L370 L371 L372 L373 | L374 L375 L376 L377 L378 L379 L380 L381 L382 L383 L384 L385 | L386 L387 L388 L389 L390 L391 L392 L393 L394 L395 L396 L397 | L398 L399 L400 L401 L402 L403 L404 L405 L406 L407 L408 L409 | L410 L411 L412 L413 L414 L415 L416 L417 L418 L419 L420 L421 | L422 L423 L424 L425 L426 L427 L428 L429 L430 L431 L432 L433 L434 L435 L436 L437 L438 L439 L440 L441 L442 L443 L444 L445 L446 L447 L448 L449 L450 L451 L452 L453 L454 L455 L456 L457 L458 L459 L460 L461 L462 L463 L464 L465 L466 L467 L468 L469 L470 L471 L472 L473 | L474 L475 L476 L477 L478 L479 L480 L481 L482 L483 L484 L485 L486 L487 L488 L489 L490 L491 L492 L493 L494 L495 L496 L497 L498 L499 L500 L501 L502 L503 L504 L505 L506 L507 L508 L509 L510 L511 L512 L513 L514 L515 L516 L517 L518 L519 L520 L521 L522 L523 L524 L525 | L526 L527 L528 L529 L530 L531 L532 L533 L534 L535 L536 L537 | L538 L539 L540 L541 L542 L543 L544 L545 L546 L547 L548 L549 | L550 L551 L552 L553 L554 L555 L556 L557 L558 L559 L560 L561 | L562 L563 L564 L565 L566 L567 L568 L569 L570 L571 L572 L573 | L574 L575 L576 L577 L578 L579 L580 L581 L582 L583 L584 L585 | L586 L587 L588 L589 L590 L591 L592 L593 L594 L595 L596 L597 | L598 L599 L600 L601 L602 L603 L604 L605 L606 L607 L608 L609 | L610 L611 L612 L613 L614 L615 L616 L617 L618 L619 L620 L621 | L622 L623 L624 L625 L626 L627 L628 L629 L630 L631 L632 L633 | L634 A9 L635 A10 L636 A11 L637 A12 picked at (-100.903597, 9.8867) picked at (-41.277767, 14.1531) picked at (-31.752767, 33.203133) picked at (-56.938431, -7.42177) picked at (-89.751843, 6.372223) picked at (-111.127454, -5.087) picked at (111.123667, 14.1531) picked at (62.344568, -6.465286) picked at (103.979667, 47.986767) picked at (106.36, 33.203133) picked at (77.785, 52.253133) picked at (92.073667, 14.1531) picked at (82.548667, 33.203133) picked at (91.250575, 41.99487) picked at (103.090333, -4.686467) picked at (48.416333, -5.087) picked at (18.583471, 10.086967) picked at (-105.666557, 33.203133) picked at (-108.047777, 52.253133) picked at (-87.38196, -4.896903) picked at (-65.184933, 28.936767) picked at (-86.907324, 29.137033) picked at (-22.2278, 14.1531) picked at (-10.637873, 29.137033) picked at (63.402, 47.986767) picked at (73.023667, -9.163307) picked at (73.023667, 14.1531) picked at (-69.9479, 47.986767) picked at (-74.711333, 14.1531) picked at (-60.327767, 14.1531) picked at (25.398667, 33.203133) picked at (6.348667, 33.203133) picked at (-50.8979, 47.986767) picked at (6.252, 47.986767) picked at (15.873, -6.01037) picked at (-19.9416, -6.01037) picked at (-50.801367, 33.203133) picked at (44.352, 47.986767) picked at (25.302, 47.986767) picked at (-31.8479, 47.986767) picked at (34.922333, 14.1531) picked at (-3.177667, 14.1531) picked at (63.498667, 33.203133) picked at (44.448667, 33.203133) picked at (58.640333, 9.8867) picked at (92.676754, 52.759393) makes body 3
move_body "Move2" bodies 3 to x (1, 0, 0) y (0, 1, 0) z (0, 0, 1) at (0, -9.5, 0)
sketch "Sketch10" plane through (0, 9.5, 0) normal (0, 1, 0) x (-1, 0, 0)
  arc A0 (-120.156293, -13.555101) -> (-117.156293, -16.555101) centre (-117.156293, -13.555101) ccw
  line L0 (-117.156293, -16.555101) -> (120.231, -16.555101)
  arc A1 (120.231, -16.555101) -> (123.231, -13.555101) centre (120.231, -13.555101) ccw
  line L1 (123.231, -13.555101) -> (123.231, 56.6448)
  arc A2 (123.231, 56.6448) -> (120.231, 59.6448) centre (120.231, 56.6448) ccw
  line L2 (120.231, 59.6448) -> (-117.156293, 59.6448)
  arc A3 (-117.156293, 59.6448) -> (-120.156293, 56.6448) centre (-117.156293, 56.6448) ccw
  line L3 (-120.156293, 56.6448) -> (-120.156293, -13.555101)
  arc A4 (19.339414, 19.279382) -> (17.022586, 19.279382) centre (18.181, 21.4948) ccw
  arc A5 (-11.174619, 38.365605) -> (-11.174619, 42.823995) centre (-12.306293, 40.5948) ccw
  arc A6 (-13.437968, 42.823995) -> (-13.437968, 38.365605) centre (-12.306293, 40.5948) ccw
  circle A7 centre (62.431, -5.905101) radius 2.5
  circle A8 centre (90.731, 42.8948) radius 2.5
  circle A9 centre (-90.056293, 5.844899) radius 2.5
  arc A10 (-89.429714, 42.918008) -> (-89.429714, 38.271592) centre (-88.506293, 40.5948) ccw
  arc A11 (-87.582873, 38.271592) -> (-87.582873, 42.918008) centre (-88.506293, 40.5948) ccw
  circle A12 centre (62.431, -5.905101) radius 1.5
  circle A13 centre (90.731, 42.8948) radius 1.5
  circle A14 centre (18.181, 21.4948) radius 1.5
  circle A15 centre (-12.306293, 40.5948) radius 1.5
  circle A16 centre (-88.506293, 40.5948) radius 1.5
  circle A17 centre (-90.056293, 5.844899) radius 1.5
  arc A18 (-43.156293, -8.205101) -> (-43.156293, -3.205101) centre (-43.156293, -5.705101) ccw
  circle A19 centre (-43.156293, -5.705101) radius 1.5
  dimension "d37" = 3
  dimension "d38" = 3
  dimension "d39" = 3
  dimension "d40" = 3
  dimension "d41" = 3
  dimension "d42" = 3
  dimension "d45" = 3
  constraint concentric A7 A12
  constraint concentric A8 A13
  constraint concentric A4 A14
  constraint concentric A5 A15
  constraint concentric A10 A16
  constraint concentric A9 A17
  constraint concentric A18 A19
  measures "d37" diameter of A12
  measures "d38" diameter of A13
  measures "d39" diameter of A14
  measures "d40" diameter of A15
  measures "d41" diameter of A16
  measures "d42" diameter of A17
  measures "d45" diameter of A19
extrude "Extrude6" cut sketch "Sketch10" against normal up to surface (2 mm away) contours A12 | A13 | A14 | A15 | A16 | A17 | A19 picked at (62.775312, -5.712392) picked at (90.84226, 42.407336) picked at (18.621421, 22.140779) picked at (-13.122119, 40.377858) picked at (-88.395033, 40.107336) picked at (-89.522028, 6.235815) picked at (-42.795352, -5.439536) bodies 3
fillet "Fillet2" radius 2 4 edges at (-129.231, 13.5, 65.6448) (-129.231, 13.5, -22.555101) (126.156293, 13.5, 65.6448) (126.156293, 13.5, -22.555101) on bodies 2
sketch "MicroB_case_cutout" plane through (0, 0, 0) normal (0, -1, 0) x (1, 0, 0)
  line L0 (121.156293, 60.6448) -> (-124.231, 60.6448)
  line L1 (-124.231, 60.6448) -> (-124.231, -17.555101)
  line L2 (-124.231, -17.555101) -> (121.156293, -17.555101)
  line L3 (121.156293, -17.555101) -> (121.156293, 60.6448)
  line L4 (-129.231, 63.6448) -> (-129.231, -20.555101)
  line L5 (-129.231, 48.6448) -> (-100.231, 48.6448) construction
  line L6 (-100.231, 48.6448) -> (-85.231, 48.6448)
  line L7 (-85.231, 48.6448) -> (-85.231, 60.6448)
  line L8 (124.156293, 65.6448) -> (-127.231, 65.6448)
  line L9 (-85.231, 60.6448) -> (-85.231, 65.6448)
  line L10 (-100.231, 48.6448) -> (-100.231, 65.6448)
  dimension "d47" = 29
  dimension "d48" = 15
  dimension "d49" = 12
  constraint coincident L4 L5.start
  constraint perpendicular L1 L5
  constraint horizontal L6
  constraint coincident L0 L7.end
  constraint coincident L8 L9.end
  constraint perpendicular L0 L9
  constraint coincident L8 L10.end
  constraint vertical L7
  constraint vertical L10
  measures "d47" distance of L5.start L5.end
  measures "d48" distance of L5.end L6.end
  measures "d49" vertical distance of L6.end L7.end
extrude "Extrude7" cut sketch "MicroB_case_cutout" against normal blind 12 contours L0 L6 L7 L10 | L0 L8 L9 L10 picked at (-95.231, 52.6448) picked at (-90.231, 62.311467) bodies 2
sketch "Sketch12" plane through (0, 9.5, 0) normal (0, 1, 0) x (-1, 0, 0)
  circle A0 centre (62.431, -5.905101) radius 1.5
  circle A1 centre (-90.056293, 5.844899) radius 1.5
  circle A2 centre (18.181, 21.4948) radius 1.5
  circle A3 centre (90.731, 42.8948) radius 1.5
  circle A4 centre (-88.506293, 40.5948) radius 1.5
  circle A5 centre (-12.306293, 40.5948) radius 1.5
  circle A6 centre (-43.156293, -5.705101) radius 1.5
  arc A7 (-120.156293, -13.555101) -> (-117.156293, -16.555101) centre (-117.156293, -13.555101) ccw
  line L0 (-117.156293, -16.555101) -> (120.231, -16.555101)
  arc A8 (120.231, -16.555101) -> (123.231, -13.555101) centre (120.231, -13.555101) ccw
  line L1 (123.231, -13.555101) -> (123.231, 56.6448)
  arc A9 (123.231, 56.6448) -> (120.231, 59.6448) centre (120.231, 56.6448) ccw
  line L2 (120.231, 59.6448) -> (-117.156293, 59.6448)
  arc A10 (-117.156293, 59.6448) -> (-120.156293, 56.6448) centre (-117.156293, 56.6448) ccw
  line L3 (-120.156293, 56.6448) -> (-120.156293, -13.555101)
  line L4 (-66.970682, -13.729026) -> (5.679311, -13.729026) construction
  line L5 (5.679311, -13.729026) -> (5.679311, 36.270974) construction
  line L6 (5.679311, 36.270974) -> (-66.970682, 36.270974) construction
  line L7 (-66.970682, 36.270974) -> (-66.970682, -13.729026) construction
  constraint perpendicular L4 L5
  constraint parallel L4 L6
  constraint parallel L5 L7
sketch "Sketch13" plane through (0, 7.5, 0) normal (0, -1, 0) x (1, 0, 0)
  circle A0 centre (-62.431, -5.905101) radius 1.5
  circle A1 centre (90.056293, 5.844899) radius 1.5
  circle A2 centre (-18.181, 21.4948) radius 1.5
  circle A3 centre (-90.731, 42.8948) radius 1.5
  circle A4 centre (88.506293, 40.5948) radius 1.5
  circle A5 centre (12.306293, 40.5948) radius 1.5
  circle A6 centre (43.156293, -5.705101) radius 1.5
  arc A7 (117.156293, -16.555101) -> (120.156293, -13.555101) centre (117.156293, -13.555101) ccw
  line L0 (120.156293, -13.555101) -> (120.156293, 56.6448)
  arc A8 (120.156293, 56.6448) -> (117.156293, 59.6448) centre (117.156293, 56.6448) ccw
  line L1 (117.156293, 59.6448) -> (-120.231, 59.6448)
  arc A9 (-120.231, 59.6448) -> (-123.231, 56.6448) centre (-120.231, 56.6448) ccw
  line L2 (-123.231, 56.6448) -> (-123.231, -13.555101)
  arc A10 (-123.231, -13.555101) -> (-120.231, -16.555101) centre (-120.231, -13.555101) ccw
  line L3 (-120.231, -16.555101) -> (117.156293, -16.555101)
  line L4 (114.656293, 59.6448) -> (114.656293, 5.6448) construction
  line L5 (114.656293, 5.6448) -> (120.156293, 5.6448) construction
  line L6 (114.656293, 5.6448) -> (117.406293, 5.6448)
  line L7 (117.406293, 5.6448) -> (117.406293, 8.87195)
  line L8 (117.406293, 8.87195) -> (114.656293, 8.87195)
  line L9 (114.656293, 8.87195) -> (114.656293, 5.6448)
  dimension "d52" = 54
  dimension "d53" = 5.5
  constraint vertical L4
  constraint horizontal L5
  constraint horizontal L6
  constraint vertical L7
  constraint horizontal L8
  constraint vertical L9
extrude "Extrude8" add sketch "Sketch13" along normal blind 1 contours L6 L7 L8 L9 picked at (115.57296, 7.796234) bodies 3
sketch "Sketch14" plane through (0, 6.5, 0) normal (0, -1, 0) x (1, 0, 0)
  line L0 (114.656293, 8.87195) -> (114.656293, 5.6448)
  line L1 (114.656293, 5.6448) -> (117.406293, 5.6448)
  line L2 (117.406293, 5.6448) -> (117.406293, 8.87195)
  line L3 (117.406293, 8.87195) -> (114.656293, 8.87195)
  circle A0 centre (116.031293, 7.258375) radius 0.821801
extrude "Extrude9" add sketch "Sketch14" along normal blind 1 contours A0 picked at (115.860499, 6.882719) bodies 3
sketch "Sketch15" plane through (0, 7.5, 0) normal (0, -1, 0) x (1, 0, 0)
  line L0 (114.656293, 8.87195) -> (117.406293, 8.87195)
  line L1 (117.406293, 8.87195) -> (117.406293, 5.6448)
  line L2 (117.406293, 5.6448) -> (114.656293, 5.6448)
  line L3 (114.656293, 5.6448) -> (114.656293, 8.87195)
  circle A0 centre (-62.431, -5.905101) radius 1.5
  circle A1 centre (90.056293, 5.844899) radius 1.5
  circle A2 centre (-18.181, 21.4948) radius 1.5
  circle A3 centre (-90.731, 42.8948) radius 1.5
  circle A4 centre (88.506293, 40.5948) radius 1.5
  circle A5 centre (12.306293, 40.5948) radius 1.5
  circle A6 centre (43.156293, -5.705101) radius 1.5
  arc A7 (117.156293, -16.555101) -> (120.156293, -13.555101) centre (117.156293, -13.555101) ccw
  line L4 (120.156293, -13.555101) -> (120.156293, 56.6448)
  arc A8 (120.156293, 56.6448) -> (117.156293, 59.6448) centre (117.156293, 56.6448) ccw
  line L5 (117.156293, 59.6448) -> (-120.231, 59.6448)
  arc A9 (-120.231, 59.6448) -> (-123.231, 56.6448) centre (-120.231, 56.6448) ccw
  line L6 (-123.231, 56.6448) -> (-123.231, -13.555101)
  arc A10 (-123.231, -13.555101) -> (-120.231, -16.555101) centre (-120.231, -13.555101) ccw
  line L7 (-120.231, -16.555101) -> (117.156293, -16.555101)
  line L8 (-89.391, 59.6448) -> (-97.391, 59.6448)
  line L9 (-97.391, 59.6448) -> (-97.391, 50.1448)
  line L10 (-97.391, 50.1448) -> (-89.391, 50.1448)
  line L11 (-89.391, 50.1448) -> (-89.391, 59.6448)
  line L12 (-89.391, 50.1448) -> (-123.231, 50.089119)
  dimension "d58" = 33.84
  dimension "d59" = 8
  dimension "d60" = 9.5
  constraint horizontal L8
  constraint vertical L9
  constraint horizontal L10
  constraint vertical L11
  constraint coincident L5 L8.start
  measures "d59" distance of L8.start L8.end
  measures "d60" distance of L8.start L10.end
extrude "Extrude10" add sketch "Sketch15" along normal blind 4 contours L5 L8 L9 L10 L11 picked at (-94.724333, 56.478133) bodies 3